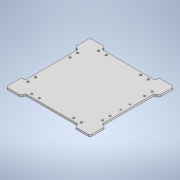
# Autodesk Inventor part: bottom_plate
Saved by Autodesk Inventor 2021 (Build 250183000, 183)
## iProperties
Created: 2020-07-18
Part Number: bottom_plate
Material: Generic
Document SubType Name: Modeling
Designer: Andrew
Density: 1 g/cm^3
Appearance: Default
Author: Andrew
Autodesk Inventor part; units mm, degrees
ref_plane "YZ Plane" through (0, 0, 0) normal (1, 0, 0) x (0, 1, 0)
ref_plane "XZ Plane" through (0, 0, 0) normal (0, 1, 0) x (-1, 0, 0)
sketch "Sketch1" plane through (0, 0, 0) normal (0, 1, 0) x (-1, 0, 0)
  line L0 (0, 0) -> (200, 0)
  line L1 (200, 0) -> (200, -200)
  line L2 (200, -200) -> (0, -200)
  line L3 (0, -200) -> (0, 0)
  dimension "d0" = 200
  dimension "d1" = 200
  constraints: 8 end point, 2 parallel, 1 horizontal, 1 perpendicular
  measures "d0" distance of L1.end L2.end
  measures "d1" distance of L0.end L1.end
extrude "Extrusion1" add sketch "Sketch1" along normal blind 5
sketch "Sketch3" plane through (0, 5, 0) normal (0, 1, 0) x (1, 0, 0)
  line L0 (-200, 0) -> (0, 0) projected
  line L1 (0, 0) -> (0, 30)
  line L2 (0, 0) -> (0, 200) projected
  line L3 (0, 30) -> (10, 30)
  line L4 (10, 30) -> (10, -10)
  line L5 (10, -10) -> (-30, -10)
  line L6 (-30, -10) -> (-30, 0)
  line L7 (-30, 0) -> (0, 0)
  line L8 (-200, 0) -> (-200, 30)
  line L9 (-200, 200) -> (-200, 0) projected
  line L10 (-200, 30) -> (-210, 30)
  line L11 (-210, 30) -> (-210, -10)
  line L12 (-210, -10) -> (-170, -10)
  line L13 (-170, -10) -> (-170, 0)
  line L14 (-170, 0) -> (-200, 0)
  dimension "d20" = 30
  dimension "d21" = 10
  dimension "d22" = 40
  dimension "d23" = 40
  dimension "d24" = 30
  dimension "d25" = 10
  dimension "d26" = 40
  dimension "d27" = 40
  constraints: 24 end point, 9 perpendicular, 3 point on line, 1 collinear
  measures "d20" distance of L0.end L1.end
  measures "d21" distance of L1.end L3.end
  measures "d22" distance of L3.end L4.end
  measures "d23" distance of L4.end L5.end
  measures "d24" distance of L0.start L8.end
  measures "d25" distance of L8.end L10.end
  measures "d26" distance of L10.end L11.end
  measures "d27" distance of L11.end L12.end
extrude "Extrusion3" add sketch "Sketch3" against normal blind 5
ref_plane "Work Plane2" through (-170, 0, -100) normal (0, 0, 1) x (1, 0, 0)
mirror "Mirror2" about plane through (-170, 0, -100) normal (0, 0, 1) of "Extrusion3"
sketch "Sketch4" plane through (0, 5, 0) normal (0, 1, 0) x (1, 0, 0)
  circle A0 centre (-7.5, 40) radius 2.5
  circle A1 centre (-7.5, 60) radius 2.5
  circle A2 centre (-30, 7.5) radius 2.5
  circle A3 centre (-50, 7.5) radius 2.5
  line L0 (-30, -10) -> (10, -10) projected
  line L1 (0, 30) -> (0, 170) projected
  line L2 (10, -10) -> (10, 30) projected
  line L3 (-170, 0) -> (-30, 0) projected
  circle A4 centre (-140, 7.5) radius 2.5
  circle A5 centre (-160, 7.5) radius 2.5
  circle A6 centre (-192.5, 30) radius 2.5
  circle A7 centre (-192.5, 50) radius 2.5
  line L4 (-210, 30) -> (-210, -10) projected
  line L5 (-210, -10) -> (-170, -10) projected
  line L6 (-200, 170) -> (-200, 30) projected
  circle A8 centre (-192.5, 160) radius 2.5
  circle A9 centre (-192.5, 140) radius 2.5
  circle A10 centre (-170, 192.5) radius 2.5
  circle A11 centre (-150, 192.5) radius 2.5
  circle A12 centre (-60, 192.5) radius 2.5
  circle A13 centre (-40, 192.5) radius 2.5
  circle A14 centre (-7.5, 170) radius 2.5
  circle A15 centre (-7.5, 150) radius 2.5
  line L7 (-30, 200) -> (-170, 200) projected
  line L8 (-30, 210) -> (10, 210) projected
  line L9 (10, 210) -> (10, 170) projected
  line L10 (-210, 170) -> (-210, 210) projected
  line L11 (-210, 210) -> (-170, 210) projected
  point P0 (0, 0)
  dimension "d30" = 5
  dimension "d31" = 5
  dimension "d32" = 5
  dimension "d33" = 5
  dimension "d34" = 70
  dimension "d35" = 50
  dimension "d36" = 7.5
  dimension "d37" = 7.5
  dimension "d38" = 40
  dimension "d39" = 60
  dimension "d40" = 7.5
  dimension "d41" = 7.5
  dimension "d42" = 5
  dimension "d43" = 5
  dimension "d44" = 5
  dimension "d45" = 5
  dimension "d46" = 50
  dimension "d47" = 70
  dimension "d48" = 40
  dimension "d49" = 60
  dimension "d50" = 7.5
  dimension "d51" = 7.5
  dimension "d52" = 7.5
  dimension "d53" = 7.5
  dimension "d123" = 7.5
  dimension "d124" = 7.5
  dimension "d125" = 7.5
  dimension "d126" = 7.5
  dimension "d127" = 7.5
  dimension "d128" = 7.5
  dimension "d129" = 7.5
  dimension "d130" = 7.5
  dimension "d131" = 5
  dimension "d132" = 5
  dimension "d133" = 5
  dimension "d134" = 5
  dimension "d135" = 5
  dimension "d136" = 5
  dimension "d137" = 5
  dimension "d138" = 5
  dimension "d139" = 40
  dimension "d140" = 60
  dimension "d141" = 50
  dimension "d142" = 70
  dimension "d143" = 40
  dimension "d144" = 60
  dimension "d145" = 50
  dimension "d146" = 70
  constraints: 16 centre point
  measures "d30" diameter of A0
  measures "d31" diameter of A1
  measures "d32" diameter of A2
  measures "d33" diameter of A3
  measures "d34" distance from line of L0 A1.centre
  measures "d35" distance from line of L0 A0.centre
  measures "d36" distance from line of L1 A0.centre
  measures "d37" distance from line of L1 A1.centre
  measures "d38" distance from line of L2 A2.centre
  measures "d39" distance from line of L2 A3.centre
  measures "d40" distance from line of L3 A2.centre
  measures "d41" distance from line of L3 A3.centre
  measures "d42" diameter of A4
  measures "d43" diameter of A5
  measures "d44" diameter of A6
  measures "d45" diameter of A7
  measures "d46" distance from line of L4 A5.centre
  measures "d47" distance from line of L4 A4.centre
  measures "d48" distance from line of L5 A6.centre
  measures "d49" distance from line of L5 A7.centre
  measures "d50" distance from line of L6 A7.centre
  measures "d51" distance from line of L6 A6.centre
  measures "d52" distance from line of L3 A5.centre
  measures "d53" distance from line of L3 A4.centre
  measures "d123" distance from line of L6 A9.centre
  measures "d124" distance from line of L6 A8.centre
  measures "d125" distance from line of L7 A10.centre
  measures "d126" distance from line of L7 A11.centre
  measures "d127" distance from line of L7 A12.centre
  measures "d128" vertical distance of L7.start A13.centre
  measures "d129" distance from line of L1 A14.centre
  measures "d130" distance from line of L1 A15.centre
  measures "d131" diameter of A9
  measures "d132" diameter of A8
  measures "d133" diameter of A10
  measures "d134" diameter of A11
  measures "d135" diameter of A12
  measures "d136" diameter of A13
  measures "d137" diameter of A14
  measures "d138" diameter of A15
  measures "d139" distance from line of A14.centre L8
  measures "d140" distance from line of A15.centre L8
  measures "d141" distance from line of A13.centre L9
  measures "d142" distance from line of A12.centre L9
  measures "d143" distance from line of A10.centre L10
  measures "d144" distance from line of A11.centre L10
  measures "d145" distance from line of L11 A8.centre
  measures "d146" distance from line of L11 A9.centre
extrude "Extrusion4" cut sketch "Sketch4" against normal through all
fillet "Fillet2" radius 5 20 edges at (-30, 2.5, 0) (-30, 2.5, 10) (10, 2.5, 10) (10, 2.5, -30) (0, 2.5, -170) (10, 2.5, -170) (0, 2.5, -30) (10, 2.5, -210) (-30, 2.5, -210) (-30, 2.5, -200) (-170, 2.5, -210) (-210, 2.5, -210) (-210, 2.5, -170) (-170, 2.5, -200) (-200, 2.5, -170) (-210, 2.5, 10) (-210, 2.5, -30) (-200, 2.5, -30) (-170, 2.5, 0) (-170, 2.5, 10)
sketch "Sketch6" plane through (0, 0, 0) normal (0, -1, 0) x (1, 0, 0)
  line L0 (-151, -40) -> (-50, -40)
  line L1 (-50, -40) -> (-50, -91)
  line L2 (-50, -91) -> (-151, -91)
  line L3 (-151, -91) -> (-151, -40)
  line L4 (-50, -99) -> (-50, -150)
  line L5 (-50, -150) -> (-121, -150)
  line L6 (-121, -150) -> (-121, -99)
  line L7 (0, -35) -> (0, -165) projected
  line L8 (-35, -200) -> (-165, -200) projected
  line L9 (-200, -165) -> (-200, -35) projected
  line L10 (-156, -35) -> (-45, -35)
  line L11 (-45, -35) -> (-45, -96)
  line L12 (-126, -96) -> (-156, -96)
  line L13 (-156, -96) -> (-156, -35)
  line L14 (-45, -155) -> (-126, -155)
  line L15 (-126, -155) -> (-126, -94)
  line L16 (-45, -94) -> (-45, -155)
  line L17 (-126, -107) -> (-121, -107)
  line L18 (-113, -94) -> (-113, -99)
  line L19 (-58, -94) -> (-58, -99)
  line L20 (-50, -107) -> (-45, -107)
  line L21 (-50, -142) -> (-45, -142)
  line L22 (-58, -150) -> (-58, -155)
  line L23 (-113, -150) -> (-113, -155)
  line L24 (-121, -142) -> (-126, -142)
  line L25 (-143, -91) -> (-143, -96)
  line L26 (-151, -83) -> (-156, -83)
  line L27 (-151, -48) -> (-156, -48)
  line L28 (-143, -35) -> (-143, -40)
  line L29 (-58, -35) -> (-58, -40)
  line L30 (-50, -48) -> (-45, -48)
  line L31 (-50, -83) -> (-45, -83)
  line L32 (-58, -91) -> (-58, -94)
  line L33 (-121, -99) -> (-113, -99)
  line L34 (-58, -99) -> (-50, -99)
  line L35 (-126, -94) -> (-113, -94)
  point P0 (0, 0)
  dimension "d57" = 50
  dimension "d58" = 101
  dimension "d59" = 50
  dimension "d61" = 51
  dimension "d62" = 79
  dimension "d63" = 51
  dimension "d64" = 5
  dimension "d65" = 5
  dimension "d66" = 5
  dimension "d68" = 5
  dimension "d69" = 5
  dimension "d70" = 5
  dimension "d71" = 5
  dimension "d73" = 8
  dimension "d74" = 8
  dimension "d75" = 8
  dimension "d76" = 8
  dimension "d77" = 8
  dimension "d78" = 8
  dimension "d79" = 8
  dimension "d80" = 8
  dimension "d81" = 8
  dimension "d82" = 8
  dimension "d84" = 8
  dimension "d85" = 8
  dimension "d86" = 8
  dimension "d87" = 8
  dimension "d88" = 104
  dimension "d89" = 101
  dimension "d90" = 106
  dimension "d91" = 93
  dimension "d92" = 93
  dimension "d93" = 106
  dimension "d94" = 104
  dimension "d95" = 106
  dimension "d96" = 106
  constraints: 66 end point, 29 point on line, 23 perpendicular, 9 parallel, 5 horizontal
  measures "d57" distance between parallel lines of L7 L1
  measures "d58" distance of L0.start L0.end
  measures "d59" distance between parallel lines of L8 L5
  measures "d61" distance of L4.start L4.end
  measures "d62" distance between parallel lines of L9 L6
  measures "d63" distance of L0.end L1.end
  measures "d64" distance between parallel lines of L16 L4
  measures "d65" distance between parallel lines of L5 L14
  measures "d66" distance between parallel lines of L6 L15
  measures "d68" distance between parallel lines of L2 L12
  measures "d69" distance between parallel lines of L3 L13
  measures "d70" distance between parallel lines of L10 L0
  measures "d71" distance between parallel lines of L11 L1
  measures "d73" distance between parallel lines of L1 L29
  measures "d74" distance between parallel lines of L0 L30
  measures "d75" distance between parallel lines of L2 L31
  measures "d76" distance between parallel lines of L1 L32
  measures "d77" distance between parallel lines of L3 L28
  measures "d78" distance between parallel lines of L0 L27
  measures "d79" distance between parallel lines of L2 L26
  measures "d80" distance between parallel lines of L3 L25
  measures "d81" distance between parallel lines of L6 L18
  measures "d82" distance between parallel lines of L4 L19
  measures "d84" distance between parallel lines of L5 L21
  measures "d85" distance between parallel lines of L4 L22
  measures "d86" distance between parallel lines of L6 L23
  measures "d87" distance between parallel lines of L5 L24
  measures "d88" distance between parallel lines of L8 L12
  measures "d89" distance between parallel lines of L8 L33
  measures "d90" distance between parallel lines of L8 L35
  measures "d91" distance between parallel lines of L8 L17
  measures "d92" distance between parallel lines of L20 L8
  measures "d93" distance from line of L16.start L8
  measures "d94" distance from line of L11.end L8
  measures "d95" distance from line of L32.end L8
  measures "d96" distance from line of L19.start L8
extrude "Extrusion5" add sketch "Sketch6" along normal blind 10 contours L3 L27 L13 L10 L28 L0 | L29 L10 L11 L30 L1 L0 | L3 L2 L25 L12 L13 L26 | L31 L11 L16 L20 L4 L34 L19 L32 L2 L1 | L15 L35 L18 L33 L6 L17 | L24 L6 L5 L23 L14 L15 | L16 L14 L22 L5 L4 L21
sketch "Sketch8" plane through (0, 0, 0) normal (0, -1, 0) x (1, 0, 0)
  line L0 (-165, 0) -> (-35, 0) projected
  line L1 (0, -35) -> (0, -165) projected
  point P0 (0, 0)
  point P1 (-7.5, -112)
  point P2 (-7.5, -88)
  dimension "d110" = 24
  dimension "d111" = 88
  dimension "d112" = 7.5
  dimension "d113" = 7.5
  measures "d110" distance of point (-7.5, -88) point (-7.5, -112)
  measures "d111" distance from line of L0 point (-7.5, -88)
  measures "d112" distance from line of L1 point (-7.5, -88)
  measures "d113" distance from line of L1 point (-7.5, -112)
hole "Hole2" at (-7.5, 0, -112) at (-7.5, 0, -88) direction (0, 1, 0) diameter 4 end through all
body "Solid1"
